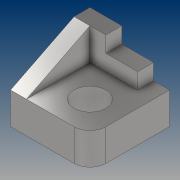
# Autodesk Inventor part: 26
Saved by Autodesk Inventor 2020.2 (Build 242310000, 310)
## iProperties
Created: 2020-09-17
Part Number: 26
Material: 鋼、碳鋼
Document SubType Name: Modeling
Designer: user
Density: 7.85 g/cm^3
Appearance: 半拋光
Mass: 418.308 g
Surface Area: 117.468 cm^2
Volume: 53.2876 cm^3
Author: user
Autodesk Inventor part; units mm, degrees
ref_plane "YZ Plane" through (0, 0, 0) normal (1, 0, 0) x (0, 1, 0)
ref_plane "XZ Plane" through (0, 0, 0) normal (0, 1, 0) x (-1, 0, 0)
ref_plane "XY Plane" through (0, 0, 0) normal (0, 0, 1) x (1, 0, 0)
sketch "草圖1" plane through (0, 0, 0) normal (0, 1, 0) x (-1, 0, 0)
  line L0 (0, 0) -> (-50, 0)
  line L1 (-50, 0) -> (-50, 50)
  line L2 (-50, 50) -> (0, 50)
  line L3 (0, 50) -> (0, 0)
  dimension "d0" = 50
  dimension "d1" = 50
  constraints: 8 end point, 2 parallel, 1 horizontal, 1 perpendicular
  measures "d0" distance of L1.end L2.end
  measures "d1" distance of L0.end L1.end
extrude "擠出1" add sketch "草圖1" along normal blind 20
fillet "圓角1" radius 10 1 edges at (50, 10, 50)
sketch "草圖2" plane through (50, 0, 0) normal (0, 0, -1) x (-1, 0, 0)
  line L0 (0, 20) -> (50, 20) projected
  line L1 (50, 20) -> (50, 0) projected
  line L2 (50, 0) -> (0, 0) projected
  line L3 (0, 0) -> (0, 20) projected
  line L4 (50, 20) -> (50, 40)
  line L5 (50, 40) -> (30, 40)
  line L6 (30, 40) -> (30, 30)
  line L7 (30, 30) -> (10, 30)
  line L8 (10, 30) -> (10, 20)
  dimension "d5" = 10
  dimension "d6" = 20
  dimension "d7" = 10
  dimension "d8" = 20
  constraints: 10 end point, 4 perpendicular, 1 point on line, 1 vertical
  measures "d5" distance between parallel lines of L3 L8
  measures "d6" distance of L4.end L5.end
  measures "d7" distance between parallel lines of L7 L0
  measures "d8" distance between parallel lines of L0 L5
extrude "擠出2" add sketch "草圖2" against normal blind 10 contours L8 L7 L6 L5 L4 L0
sketch "草圖3" plane through (0, 0, 0) normal (-1, 0, 0) x (0, 0, 1)
  line L0 (0, 40) -> (10, 40) projected
  line L1 (10, 40) -> (10, 20) projected
  line L2 (10, 20) -> (50, 20) projected
  line L3 (50, 20) -> (50, 0) projected
  line L4 (50, 0) -> (0, 0) projected
  line L5 (0, 0) -> (0, 40) projected
  line L6 (10, 40) -> (10, 20) projected
  line L7 (40, 20) -> (50, 20) projected
  line L8 (10, 40) -> (50, 20)
  constraints: 2 end point
extrude "擠出3" add sketch "草圖3" against normal blind 10 contours L8 L2 L1
sketch "草圖4" plane through (0, 20, 0) normal (0, 1, 0) x (1, 0, 0)
  arc A0 (40, -50) -> (50, -40) centre (40, -40) ccw projected
  line L0 (40, -50) -> (10, -50) projected
  line L1 (10, -10) -> (10, -50) projected
  line L2 (40, -10) -> (10, -10) projected
  line L3 (40, 0) -> (40, -10) projected
  line L4 (0, 0) -> (40, 0) projected
  line L5 (0, -50) -> (0, 0) projected
  line L6 (10, -50) -> (0, -50) projected
  line L7 (50, 0) -> (50, -40) projected
  line L8 (40, 0) -> (50, 0) projected
  circle A1 centre (30, -30) radius 10
  dimension "d13" = 20
  dimension "d14" = 20
  dimension "d15" = 20
  constraints: 1 centre point
  measures "d13" distance from line of L7 A1.centre
  measures "d14" distance from line of L0 A1.centre
  measures "d15" diameter of A1
extrude "擠出4" cut sketch "草圖4" against normal through all contours A1
